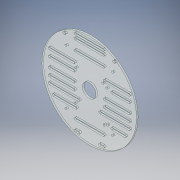
# Autodesk Inventor part: Part1-Estructura grande
Saved by Autodesk Inventor 2019 (Build 230136000, 136)
## iProperties
Created: 2023-04-24
Part Number: Part1-Estructura grande
Material: Generic
Document SubType Name: Modeling
Designer: Tecneu Technology
Density: 1 g/cm^3
Appearance: Glazing
Author: Tecneu Technology
Autodesk Inventor part; units mm, degrees
ref_plane "YZ Plane" through (0, 0, 0) normal (1, 0, 0) x (0, 1, 0)
ref_plane "XZ Plane" through (0, 0, 0) normal (0, 1, 0) x (-1, 0, 0)
ref_plane "XY Plane" through (0, 0, 0) normal (0, 0, 1) x (1, 0, 0)
sketch "Sketch1" plane through (0, 0, 0) normal (0, 0, 1) x (1, 0, 0)
  circle A0 centre (0, 0) radius 70
  circle A1 centre (0, 0) radius 10.082
  line L0 (-1.672, 60.8463) -> (-20.9127, 60.8463)
  line L1 (-20.9127, 64.1904) -> (-1.672, 64.1904)
  arc A2 (-20.9127, 64.1904) -> (-20.9127, 60.8463) centre (-20.9127, 62.5184) ccw
  line L2 (-1.672, 64.1904) -> (0, 64.1904)
  line L3 (-1.672, 60.8463) -> (0, 60.8463)
  line L4 (1.672, 60.8463) -> (20.9127, 60.8463)
  line L5 (20.9127, 64.1904) -> (1.672, 64.1904)
  arc A3 (20.9127, 60.8463) -> (20.9127, 64.1904) centre (20.9127, 62.5184) ccw
  line L6 (1.672, 64.1904) -> (0, 64.1904)
  line L7 (1.672, 60.8463) -> (0, 60.8463)
  line L8 (-1.672, 54.4078) -> (-20.9127, 54.4078)
  line L9 (-20.9127, 57.7519) -> (-1.672, 57.7519)
  arc A4 (-20.9127, 57.7519) -> (-20.9127, 54.4078) centre (-20.9127, 56.0799) ccw
  line L10 (-1.672, 57.7519) -> (0, 57.7519)
  line L11 (-1.672, 54.4078) -> (0, 54.4078)
  line L12 (1.672, 54.4078) -> (20.9127, 54.4078)
  line L13 (20.9127, 57.7519) -> (1.672, 57.7519)
  arc A5 (20.9127, 54.4078) -> (20.9127, 57.7519) centre (20.9127, 56.0799) ccw
  line L14 (1.672, 54.4078) -> (0, 54.4078)
  line L15 (1.672, 57.7519) -> (0, 57.7519)
  line L16 (-1.672, 39.0652) -> (-20.9127, 39.0652)
  line L17 (-20.9127, 42.4093) -> (-1.672, 42.4093)
  arc A6 (-20.9127, 42.4093) -> (-20.9127, 39.0652) centre (-20.9127, 40.7373) ccw
  line L18 (-1.672, 42.4093) -> (0, 42.4093)
  line L19 (-1.672, 39.0652) -> (0, 39.0652)
  line L20 (1.672, 39.0652) -> (20.9127, 39.0652)
  line L21 (20.9127, 42.4093) -> (1.672, 42.4093)
  arc A7 (20.9127, 39.0652) -> (20.9127, 42.4093) centre (20.9127, 40.7373) ccw
  line L22 (1.672, 39.0652) -> (0, 39.0652)
  line L23 (1.672, 42.4093) -> (0, 42.4093)
  line L24 (-1.672, -48.5783) -> (-20.9127, -48.5783)
  line L25 (-1.672, -48.5783) -> (0, -48.5783)
  line L26 (1.672, -48.5783) -> (20.9127, -48.5783)
  line L27 (1.672, -48.5783) -> (0, -48.5783)
  arc A8 (20.9127, -48.5783) -> (20.9127, -45.2342) centre (20.9127, -46.9062) ccw
  line L28 (20.9127, -45.2342) -> (1.672, -45.2342)
  line L29 (1.672, -45.2342) -> (0, -45.2342)
  line L30 (-1.672, -45.2342) -> (0, -45.2342)
  line L31 (-20.9127, -45.2342) -> (-1.672, -45.2342)
  arc A9 (-20.9127, -45.2342) -> (-20.9127, -48.5783) centre (-20.9127, -46.9062) ccw
  line L32 (-15.5223, -63.7012) -> (-20.9127, -63.7012)
  line L33 (-20.9127, -60.3572) -> (-15.5223, -60.3572)
  arc A10 (-20.9127, -60.3572) -> (-20.9127, -63.7012) centre (-20.9127, -62.0292) ccw
  arc A11 (-15.5223, -63.7012) -> (-15.5223, -60.3572) centre (-15.5223, -62.0292) ccw
  line L34 (15.5223, -63.7012) -> (20.9127, -63.7012)
  arc A12 (20.9127, -63.7012) -> (20.9127, -60.3572) centre (20.9127, -62.0292) ccw
  line L35 (20.9127, -60.3572) -> (15.5223, -60.3572)
  arc A13 (15.5223, -60.3572) -> (15.5223, -63.7012) centre (15.5223, -62.0292) ccw
  line L36 (36.2353, 53.4096) -> (37.4232, 53.4096)
  line L37 (34.5633, 55.0816) -> (34.5633, 55.0816)
  line L38 (36.2353, 56.7537) -> (37.4232, 56.7537)
  line L39 (39.0952, 55.0816) -> (39.0952, 55.0816)
  arc A14 (36.2353, 56.7537) -> (34.5633, 55.0816) centre (36.2353, 55.0816) ccw
  arc A15 (34.5633, 55.0816) -> (36.2353, 53.4096) centre (36.2353, 55.0816) ccw
  arc A16 (37.4232, 53.4096) -> (39.0952, 55.0816) centre (37.4232, 55.0816) ccw
  arc A17 (39.0952, 55.0816) -> (37.4232, 56.7537) centre (37.4232, 55.0816) ccw
  line L40 (-36.2353, 53.4096) -> (-37.4232, 53.4096)
  line L41 (-34.5633, 55.0816) -> (-34.5633, 55.0816)
  line L42 (-36.2353, 56.7537) -> (-37.4232, 56.7537)
  line L43 (-39.0952, 55.0816) -> (-39.0952, 55.0816)
  arc A18 (-34.5633, 55.0816) -> (-36.2353, 56.7537) centre (-36.2353, 55.0816) ccw
  arc A19 (-36.2353, 53.4096) -> (-34.5633, 55.0816) centre (-36.2353, 55.0816) ccw
  arc A20 (-39.0952, 55.0816) -> (-37.4232, 53.4096) centre (-37.4232, 55.0816) ccw
  arc A21 (-37.4232, 56.7537) -> (-39.0952, 55.0816) centre (-37.4232, 55.0816) ccw
  line L44 (-41.8752, -1.672) -> (-22.6346, -1.672)
  line L45 (-41.8752, -1.672) -> (-43.5472, -1.672)
  arc A22 (-22.6346, -1.672) -> (-22.6346, 1.672) centre (-22.6346, 0) ccw
  line L46 (-22.6346, 1.672) -> (-41.8752, 1.672)
  line L47 (-41.8752, 1.672) -> (-43.5472, 1.672)
  arc A23 (-59.2193, 1.672) -> (-59.2193, -1.672) centre (-59.2193, 0) ccw
  line L48 (-59.2193, 1.672) -> (-43.5472, 1.672)
  line L49 (-43.5472, -1.672) -> (-59.2193, -1.672)
  arc A24 (-22.6346, -12.0036) -> (-22.6346, -8.6595) centre (-22.6346, -10.3316) ccw
  line L50 (-22.6346, -8.6595) -> (-41.8752, -8.6595)
  line L51 (-41.8752, -12.0036) -> (-22.6346, -12.0036)
  line L52 (-41.8752, -8.6595) -> (-43.5472, -8.6595)
  line L53 (-41.8752, -12.0036) -> (-43.5472, -12.0036)
  arc A25 (-59.2193, -8.6595) -> (-59.2193, -12.0036) centre (-59.2193, -10.3316) ccw
  line L54 (-59.2193, -8.6595) -> (-43.5472, -8.6595)
  line L55 (-43.5472, -12.0036) -> (-59.2193, -12.0036)
  arc A26 (-22.6346, 12.3529) -> (-22.6346, 15.697) centre (-22.6346, 14.025) ccw
  line L56 (-22.6346, 15.697) -> (-41.8752, 15.697)
  line L57 (-41.8752, 12.3529) -> (-22.6346, 12.3529)
  line L58 (-41.8752, 15.697) -> (-43.5472, 15.697)
  line L59 (-41.8752, 12.3529) -> (-43.5472, 12.3529)
  arc A27 (-59.2193, 15.697) -> (-59.2193, 12.3529) centre (-59.2193, 14.025) ccw
  line L60 (-59.2193, 15.697) -> (-43.5472, 15.697)
  line L61 (-43.5472, 12.3529) -> (-59.2193, 12.3529)
  arc A28 (-59.2193, 26.2282) -> (-59.2193, 22.8841) centre (-59.2193, 24.5561) ccw
  line L62 (-59.2193, 26.2282) -> (-43.5472, 26.2282)
  line L63 (-43.5472, 22.8841) -> (-59.2193, 22.8841)
  line L64 (-41.8752, 22.8841) -> (-43.5472, 22.8841)
  line L65 (-41.8752, 22.8841) -> (-22.6346, 22.8841)
  arc A29 (-22.6346, 22.8841) -> (-22.6346, 26.2282) centre (-22.6346, 24.5561) ccw
  line L66 (-22.6346, 26.2282) -> (-41.8752, 26.2282)
  line L67 (-41.8752, 26.2282) -> (-43.5472, 26.2282)
  line L68 (-43.5472, -21.8959) -> (-59.2193, -21.8959)
  line L69 (-41.8752, -21.8959) -> (-43.5472, -21.8959)
  line L70 (-41.8752, -21.8959) -> (-22.6346, -21.8959)
  line L71 (-22.6346, -18.5519) -> (-41.8752, -18.5519)
  line L72 (-41.8752, -18.5519) -> (-43.5472, -18.5519)
  line L73 (-59.2193, -18.5519) -> (-43.5472, -18.5519)
  arc A30 (-59.2193, -18.5519) -> (-59.2193, -21.8959) centre (-59.2193, -20.2239) ccw
  arc A31 (-15.7718, -21.8959) -> (-15.7718, -18.5519) centre (-15.7718, -20.2239) ccw
  line L74 (-22.6346, -18.5519) -> (-15.7718, -18.5519)
  line L75 (-22.6346, -21.8959) -> (-15.7718, -21.8959)
  arc A32 (22.6346, 1.672) -> (22.6346, -1.672) centre (22.6346, 0) ccw
  line L76 (22.6346, 1.672) -> (41.8752, 1.672)
  line L77 (41.8752, -1.672) -> (22.6346, -1.672)
  line L78 (41.8752, 1.672) -> (43.5472, 1.672)
  line L79 (41.8752, -1.672) -> (43.5472, -1.672)
  arc A33 (59.2193, -1.672) -> (59.2193, 1.672) centre (59.2193, 0) ccw
  line L80 (59.2193, 1.672) -> (43.5472, 1.672)
  line L81 (43.5472, -1.672) -> (59.2193, -1.672)
  line L82 (43.5472, -12.0036) -> (59.2193, -12.0036)
  line L83 (41.8752, -12.0036) -> (43.5472, -12.0036)
  line L84 (41.8752, -12.0036) -> (22.6346, -12.0036)
  arc A34 (22.6346, -8.6595) -> (22.6346, -12.0036) centre (22.6346, -10.3316) ccw
  line L85 (22.6346, -8.6595) -> (41.8752, -8.6595)
  line L86 (41.8752, -8.6595) -> (43.5472, -8.6595)
  line L87 (59.2193, -8.6595) -> (43.5472, -8.6595)
  arc A35 (59.2193, -12.0036) -> (59.2193, -8.6595) centre (59.2193, -10.3316) ccw
  line L88 (43.5472, -21.8959) -> (59.2193, -21.8959)
  arc A36 (59.2193, -21.8959) -> (59.2193, -18.5519) centre (59.2193, -20.2239) ccw
  line L89 (59.2193, -18.5519) -> (43.5472, -18.5519)
  line L90 (22.6346, -18.5519) -> (41.8752, -18.5519)
  line L91 (41.8752, -18.5519) -> (43.5472, -18.5519)
  line L92 (41.8752, -21.8959) -> (43.5472, -21.8959)
  line L93 (41.8752, -21.8959) -> (22.6346, -21.8959)
  arc A37 (15.7718, -18.5519) -> (15.7718, -21.8959) centre (15.7718, -20.2239) ccw
  line L94 (22.6346, -18.5519) -> (15.7718, -18.5519)
  line L95 (22.6346, -21.8959) -> (15.7718, -21.8959)
  circle A38 centre (-34.4385, 40.6774) radius 1.4973
  circle A39 centre (34.4385, 40.6774) radius 1.4973
  circle A40 centre (-34.4385, -40.6774) radius 1.4973
  circle A41 centre (34.4385, -40.6774) radius 1.4973
  arc A42 (53.2299, -34.0492) -> (53.2299, -30.7052) centre (53.2299, -32.3772) ccw
  arc A43 (33.615, -30.7052) -> (33.615, -34.0492) centre (33.615, -32.3772) ccw
  line L96 (33.615, -30.7052) -> (53.2299, -30.7052)
  line L97 (33.615, -34.0492) -> (53.2299, -34.0492)
  line L98 (43.5472, 12.4528) -> (59.2193, 12.4528)
  arc A44 (59.2193, 12.4528) -> (59.2193, 15.7968) centre (59.2193, 14.1248) ccw
  line L99 (59.2193, 15.7968) -> (43.5472, 15.7968)
  line L100 (41.8752, 15.7968) -> (43.5472, 15.7968)
  line L101 (41.8752, 12.4528) -> (43.5472, 12.4528)
  arc A45 (33.615, 15.7968) -> (33.615, 12.4528) centre (33.615, 14.1248) ccw
  line L102 (33.615, 15.7968) -> (41.8752, 15.7968)
  line L103 (41.8752, 12.4528) -> (33.615, 12.4528)
  arc A46 (22.6346, 25.6392) -> (22.6346, 22.2952) centre (22.6346, 23.9672) ccw
  line L104 (41.8752, 22.2952) -> (22.6346, 22.2952)
  line L105 (22.6346, 25.6392) -> (41.8752, 25.6392)
  line L106 (43.5472, 22.2952) -> (59.2193, 22.2952)
  arc A47 (59.2193, 22.2952) -> (59.2193, 25.6392) centre (59.2193, 23.9672) ccw
  line L107 (59.2193, 25.6392) -> (43.5472, 25.6392)
  line L108 (41.8752, 25.6392) -> (43.5472, 25.6392)
  line L109 (41.8752, 22.2952) -> (43.5472, 22.2952)
  arc A48 (-53.2299, -30.7052) -> (-53.2299, -34.0492) centre (-53.2299, -32.3772) ccw
  arc A49 (-19.8446, -34.0492) -> (-19.8446, -30.7052) centre (-19.8446, -32.3772) ccw
  line L110 (-53.2299, -30.7052) -> (-19.8446, -30.7052)
  line L111 (-19.8446, -34.0492) -> (-53.2299, -34.0492)
  circle A50 centre (-21.0873, -26.887) radius 1.4973
  circle A51 centre (-19.9643, 19.2906) radius 1.4973
  circle A52 centre (19.9643, 19.2906) radius 1.4973
  circle A53 centre (25.9537, 15.8717) radius 1.4973
  circle A54 centre (21.9608, -33.3754) radius 1.4973
  circle A55 centre (26.9519, -30.8799) radius 1.4973
  point P0 (-11.2923, 62.5184)
  point P1 (11.2923, 62.5184)
  dimension "d77" = 140
  constraints: 224 end point, 88 point on circle, 56 centre point, 31 tangent, 11 horizontal, 9 parallel, 3 equal radius, 2 perpendicular, 1 coincident, 1 vertical
  measures "d77" diameter of A0
extrude "Extrusion1" add sketch "Sketch1" along normal blind 2.45
body "Solid1"
